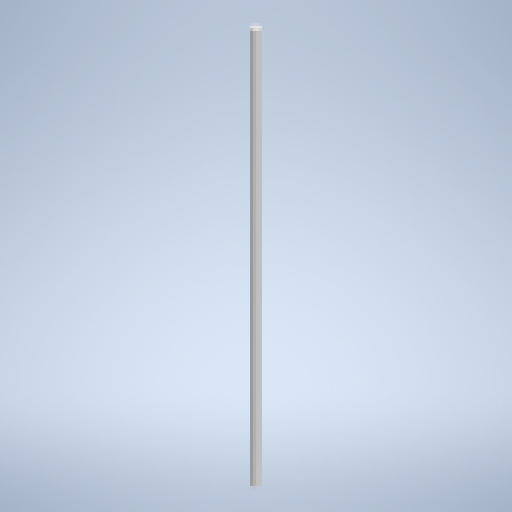
# Autodesk Inventor part: RodCenter
Saved by Autodesk Inventor 2023 (Build 270158000, 158)
## iProperties
Created: 2023-02-18
Part Number: RodCenter
Material: Stainless Steel
Document SubType Name: Modeling
Designer: phill
Density: 8 g/cm^3
Appearance: Semi-Polished
Author: phill
Autodesk Inventor part; units mm, degrees
ref_plane "YZ Plane" through (0, 0, 0) normal (1, 0, 0) x (0, 1, 0)
ref_plane "XZ Plane" through (0, 0, 0) normal (0, 1, 0) x (-1, 0, 0)
sketch "Sketch1" plane through (0, 0, 0) normal (0, 1, 0) x (-1, 0, 0)
  circle A0 centre (0, 0) radius 0.5 projected
  circle A1 centre (0, 0) radius 0.49
  point P0 (0, 0)
  dimension "d2" = 0.01
  constraints: 1 centre point
  measures "d2" radial gap between concentric circles of A0 A1
ref_plane "Work Plane1" through (-3, -48, -90) normal (0, -1, 0) x (1, 0, 0)
extrude "Extrusion1" add sketch "Sketch1" along normal blind 50 and the other way blind 50 contours A1
body "Solid1"
